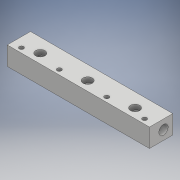
# Autodesk Inventor part: manifold
Saved by Autodesk Inventor 2018 (Build 220112000, 112)
## iProperties
Created: 2018-06-04
Part Number: manifold
Material: Generic
Document SubType Name: Modeling
Designer: John Viljoen
Density: 1 g/cm^3
Appearance: Default
Author: John Viljoen
Autodesk Inventor part; units mm, degrees
ref_plane "YZ Plane" through (0, 0, 0) normal (1, 0, 0) x (0, 1, 0)
ref_plane "XZ Plane" through (0, 0, 0) normal (0, 1, 0) x (-1, 0, 0)
ref_plane "XY Plane" through (0, 0, 0) normal (0, 0, 1) x (1, 0, 0)
sketch "Sketch1" plane through (0, 0, 0) normal (0, 0, 1) x (1, 0, 0)
  line L0 (0, 0) -> (97.04, 0)
  line L1 (97.04, 0) -> (97.04, 15.875)
  line L2 (97.04, 15.875) -> (0, 15.875)
  line L3 (0, 15.875) -> (0, 0)
  dimension "d0" = 97.04
  dimension "d1" = 15.875
  constraints: 8 end point, 2 parallel, 1 horizontal, 1 perpendicular
  measures "d0" distance of L2.end L1.end
  measures "d1" distance of L1.end L0.end
extrude "Extrusion1" add sketch "Sketch1" along normal blind 12.7
sketch "Sketch2" plane through (0, 0, 12.7) normal (0, 0, 1) x (1, 0, 0)
  line L0 (0, 0) -> (97.04, 0) projected
  line L1 (0, 15.875) -> (0, 0) projected
  line L2 (0, 0) -> (0, 6.35) construction
  line L3 (0, 6.35) -> (16.1733, 6.35) construction
  line L4 (16.1733, 6.35) -> (48.52, 6.35) construction
  line L5 (48.52, 6.35) -> (80.8667, 6.35) construction
  circle A0 centre (16.1733, 6.35) radius 3.175
  circle A1 centre (48.52, 6.35) radius 3.175
  circle A2 centre (80.8667, 6.35) radius 3.175
  circle A3 centre (32.3467, 3.175) radius 1.5
  circle A4 centre (64.6933, 3.175) radius 1.5
  line L6 (12.9983, 6.35) -> (6.4993, 6.35) construction
  line L7 (6.4993, 6.35) -> (6.4993, 3.175) construction
  line L8 (84.0417, 6.35) -> (90.5407, 6.35) construction
  line L9 (90.5407, 6.35) -> (90.5407, 3.175) construction
  circle A5 centre (6.4993, 3.175) radius 1.5
  circle A6 centre (90.5407, 3.175) radius 1.5
  dimension "d8" = 6.35
  dimension "d10" = 6.35
  dimension "d4" = 6.35
  dimension "d5" = 16.1733
  dimension "d6" = 32.3467
  dimension "d7" = 32.3467
  dimension "d9" = 6.35
  dimension "d12" = 3
  dimension "d13" = 3
  dimension "d14" = 6.499
  dimension "d15" = 6.499
  dimension "d16" = 3
  dimension "d17" = 3
  constraints: 16 end point, 5 centre point, 5 coincident, 5 point on line, 3 perpendicular, 2 horizontal alignment, 1 horizontal, 4 other
  measures "d4" distance of L0.start L2.end
  measures "d5" distance of L2.end L3.end
  measures "d6" distance of L3.end L4.end
  measures "d7" distance of L4.end L5.end
  measures "d9" diameter of A1
  measures "d12" diameter of A3
  measures "d13" diameter of A4
  measures "d14" distance of L6.start L6.end
  measures "d15" distance of L8.start L8.end
  measures "d16" diameter of A5
  measures "d17" diameter of A6
extrude "Extrusion2" cut sketch "Sketch2" against normal through all contours A3 | A4 | A5 | A6
sketch "Sketch3" plane through (0, 0, 12.7) normal (0, 0, 1) x (1, 0, 0)
  line L0 (16.1733, 6.35) -> (48.52, 6.35) construction
  line L1 (48.52, 6.35) -> (80.8667, 6.35) construction
  circle A0 centre (16.1733, 6.35) radius 3.175
  circle A1 centre (48.52, 6.35) radius 3.175
  circle A2 centre (80.8667, 6.35) radius 3.175
  point P0 (32.3467, 3.175)
  point P1 (64.6933, 3.175)
  point P2 (12.9983, 6.35)
  point P3 (84.0417, 6.35)
  dimension "d22" = 6.35
  dimension "d24" = 6.35
  dimension "d20" = 32.3467
  dimension "d21" = 32.3467
  dimension "d23" = 6.35
  constraints: 4 end point, 3 coincident, 2 horizontal alignment, 1 centre point, 1 point on line, 4 other
  measures "d20" distance of L0.start L1.start
  measures "d21" distance of L1.start L1.end
  measures "d23" diameter of A1
extrude "Extrusion3" cut sketch "Sketch3" against normal blind 9.525
sketch "Sketch4" plane through (97.04, 0, 0) normal (1, 0, 0) x (0, 0, -1)
  line L0 (-12.7, 15.875) -> (-12.7, 9.525) construction
  line L1 (-12.7, 15.875) -> (-12.7, 0) construction
  line L2 (-12.7, 9.525) -> (-6.35, 9.525) construction
  line L3 (-12.7, 9.525) -> (-3.175, 9.525) construction
  circle A0 centre (-6.35, 9.525) radius 3.175
  dimension "d27" = 6.35
  dimension "d28" = 6.35
  constraints: 4 end point, 2 point on line, 1 centre point, 1 coincident
  measures "d27" distance of L0.start L0.end
  measures "d28" diameter of A0
extrude "Extrusion4" cut sketch "Sketch4" against normal blind 84.042
body "Solid1"
